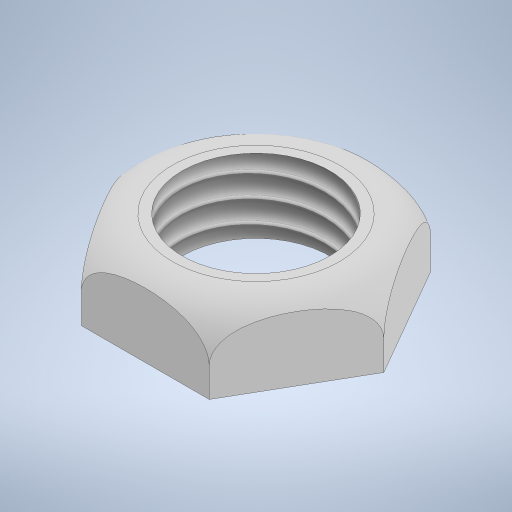
# Autodesk Inventor part: NUT
Saved by Autodesk Inventor 2023 (Build 270158000, 158)
## iProperties
Created: 2025-10-05
Part Number: NUT
Material: Generic
Document SubType Name: Modeling
Designer: ayush
Density: 1 g/cm^3
Appearance: Default
Author: ayush
Autodesk Inventor part; units mm, degrees
ref_plane "YZ Plane" through (0, 0, 0) normal (1, 0, 0) x (0, 1, 0)
ref_plane "XZ Plane" through (0, 0, 0) normal (0, 1, 0) x (-1, 0, 0)
ref_plane "XY Plane" through (0, 0, 0) normal (0, 0, 1) x (1, 0, 0)
sketch "Sketch1" plane through (0, 0, 0) normal (0, 1, 0) x (-1, 0, 0)
  line L0 (-8.6603, 0) -> (-4.3301, 7.5)
  line L1 (-4.3301, 7.5) -> (4.3301, 7.5)
  line L2 (4.3301, 7.5) -> (8.6603, 0)
  line L3 (8.6603, 0) -> (4.3301, -7.5)
  line L4 (4.3301, -7.5) -> (-4.3301, -7.5)
  line L5 (-4.3301, -7.5) -> (-8.6603, 0)
  circle A0 centre (0, 0) radius 5
  dimension "d0" = 15
  dimension "d1" = 10
  constraints: 12 end point, 2 coincident, 1 centre point, 1 horizontal alignment, 13 other
  measures "d0" distance between parallel lines of L1 L4
  measures "d1" diameter of A0
extrude "Extrusion1" add sketch "Sketch1" along normal blind 5
sketch "Sketch5" plane through (0, 0, 0) normal (0, 0, 1) x (1, 0, 0)
  line L0 (8.6603, 5) -> (4.3301, 5) projected
  line L1 (5.6603, 5) -> (8.6603, 5)
  line L2 (8.6603, 2) -> (8.6603, 2.1818)
  arc A0 (8.6603, 2) -> (5.6603, 5) centre (5.6603, 2) ccw
  line L3 (8.6603, 2) -> (8.6603, 5)
  line L4 (0, 0) -> (0, 10.7408) construction
  dimension "d6" = 3
  constraints: 9 end point, 3 tangent, 3 vertical, 2 point on circle, 1 centre point, 1 collinear, 1 point on line
  measures "d6" radius of A0
revolve "Revolution1" cut sketch "Sketch5" angle 360 about axis through (0, 0, 0) along (0, 1, 0)
thread "Thread1" size "M10x1.5" class "6H" standard "ANSI Metric M Profile" full length
body "Solid1"
